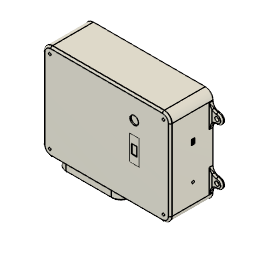
ROR Controller Housing v3 (Autodesk Fusion 360 design; units mm, degrees)
Autodesk Fusion 360 part; units mm, degrees
sketch "PCB Outline" plane through (0, 0, 0) normal (0, 0, 1) x (-1, 0, 0)
  line L0 (36.6395, 48.387) -> (-36.6395, 48.387) construction
  line L1 (-36.6395, 48.387) -> (-36.6395, -48.387) construction
  line L2 (-36.6395, -48.387) -> (36.6395, -48.387) construction
  line L3 (36.6395, -48.387) -> (36.6395, 48.387) construction
  line L4 (36.6395, 48.387) -> (-36.6395, -48.387) construction
  line L5 (-36.6395, 48.387) -> (36.6395, -48.387) construction
  line L6 (36.6395, 44.196) -> (-36.6395, 44.196) construction
  line L7 (33.5915, -48.387) -> (33.5915, 48.387) construction
  circle A0 centre (33.5915, 44.196) radius 1.5875 construction
  circle A1 centre (-32.9565, 44.196) radius 1.5875 construction
  circle A2 centre (33.5915, -44.196) radius 1.5875 construction
  circle A3 centre (-32.9565, -44.196) radius 1.5875 construction
  line L8 (-79.451, -48.75) -> (-59.451, -48.75) construction
  line L9 (-59.451, -48.75) -> (-59.451, 31.25) construction
  line L10 (-59.451, 31.25) -> (-79.451, 31.25) construction
  line L11 (-79.451, 31.25) -> (-79.451, -48.75) construction
  line L12 (-79.451, -48.75) -> (-59.451, 31.25) construction
  line L13 (-59.451, -48.75) -> (-79.451, 31.25) construction
  line L14 (-77.301, -46.625) -> (-61.601, -46.625) construction
  line L15 (-61.601, -46.625) -> (-61.601, 29.125) construction
  line L16 (-61.601, 29.125) -> (-77.301, 29.125) construction
  line L17 (-77.301, 29.125) -> (-77.301, -46.625) construction
  line L18 (-77.301, -46.625) -> (-61.601, 29.125) construction
  line L19 (-61.601, -46.625) -> (-77.301, 29.125) construction
  circle A4 centre (-77.301, -46.625) radius 1 construction
  circle A5 centre (-61.601, -46.625) radius 1 construction
  circle A6 centre (-77.301, 29.125) radius 1 construction
  circle A7 centre (-61.601, 29.125) radius 1 construction
  point P0 (-69.451, -8.75)
  point P1 (-69.451, -8.75)
  dimension "d1" = 73.279
  dimension "d2" = 96.774
  dimension "d3" = -4.191
  dimension "d4" = -3.048
  dimension "d5" = 3.175
  dimension "d8" = -66.548
  dimension "d9" = -88.392
  dimension "d11" = 70
  dimension "d12" = 20
  dimension "d13" = 80
  dimension "d14" = 15.7
  dimension "d15" = 75.75
  dimension "d16" = 2
  constraint horizontal L0
  constraint perpendicular L0 L1
  constraint parallel L0 L2
  constraint parallel L1 L3
  constraint coincident L4 origin
  constraint coincident L5 origin
  constraint coincident L7 A0.centre
  constraint coincident L6 A0.centre
  constraint horizontal L8
  constraint perpendicular L8 L9
  constraint parallel L8 L10
  constraint parallel L9 L11
  constraint coincident L12 P1
  constraint coincident L13 P1
  constraint horizontal L14
  constraint perpendicular L14 L15
  constraint parallel L14 L16
  constraint parallel L15 L17
  constraint coincident L18 P1
  constraint coincident L19 P1
  constraint coincident P1 P0
  constraint coincident L14.start L17.end
  constraint coincident L14.end L15.start
  constraint coincident L16.end L17.start
  constraint coincident L15.end L16.start
  constraint equal A4 A6
  constraint equal A4 A7
  constraint equal A4 A5
  measures "d1" distance of L1.end L2.end
  measures "d2" distance of L0.end L1.end
  measures "d5" diameter of A0
  measures "d11" distance of origin P1
  measures "d12" distance of L9.end L10.end
  measures "d13" distance of L8.end L9.end
  measures "d14" distance of L15.end L16.end
  measures "d15" distance of L14.end L15.end
  measures "d16" diameter of A4
other "Base Mesh Feature2"
other "MeshRepair2"
other "Modify2"
other "Modify3"
sketch "Base" plane through (0, 0, 0) normal (0, 0, 1) x (1, 0, 0)
  line L0 (-55, 57.5) -> (-55, -57.5)
  line L1 (-47.5, -65) -> (112.5, -65)
  line L2 (120, -57.5) -> (120, 57.5)
  line L3 (112.5, 65) -> (-47.5, 65)
  circle A0 centre (-33.5915, 44.196) radius 3.75
  circle A1 centre (32.9565, 44.196) radius 3.75
  circle A2 centre (32.9565, -44.196) radius 3.75
  circle A3 centre (-33.5915, -44.196) radius 3.75
  circle A4 centre (61.601, 46.625) radius 3.75
  circle A5 centre (77.301, 46.625) radius 3.75
  circle A6 centre (77.301, -29.125) radius 3.75
  circle A7 centre (61.601, -29.125) radius 3.75
  arc A8 (-47.5, 65) -> (-55, 57.5) centre (-47.5, 57.5) ccw
  arc A9 (120, 57.5) -> (112.5, 65) centre (112.5, 57.5) ccw
  arc A10 (112.5, -65) -> (120, -57.5) centre (112.5, -57.5) ccw
  arc A11 (-55, -57.5) -> (-47.5, -65) centre (-47.5, -57.5) ccw
  line L4 (-47.5, -68.5) -> (112.5, -68.5)
  arc A12 (112.5, -68.5) -> (123.5, -57.5) centre (112.5, -57.5) ccw
  line L5 (123.5, -57.5) -> (123.5, 57.5)
  arc A13 (123.5, 57.5) -> (112.5, 68.5) centre (112.5, 57.5) ccw
  line L6 (112.5, 68.5) -> (-47.5, 68.5)
  arc A14 (-47.5, 68.5) -> (-58.5, 57.5) centre (-47.5, 57.5) ccw
  line L7 (-58.5, 57.5) -> (-58.5, -57.5)
  arc A15 (-58.5, -57.5) -> (-47.5, -68.5) centre (-47.5, -57.5) ccw
  line L8 (-58.5, 0) -> (123.5, 0) construction
  line L9 (123.5, 0) -> (132.5, 0) construction
  line L10 (-58.5, 0) -> (-67.5, 0) construction
  line L11 (132.5, 0) -> (132.5, 40) construction
  line L12 (132.5, 0) -> (132.5, -40) construction
  line L13 (-67.5, 0) -> (-67.5, 40) construction
  line L14 (-67.5, 0) -> (-67.5, -40) construction
  circle A16 centre (-67.5, 40) radius 7.5
  circle A17 centre (-67.5, -40) radius 7.5
  circle A18 centre (132.5, -40) radius 7.5
  circle A19 centre (132.5, 40) radius 7.5
  line L15 (132.5, 32.5) -> (123.5, 32.5)
  line L16 (132.5, 47.5) -> (123.5, 47.5)
  line L17 (132.5, -32.5) -> (123.5, -32.5)
  line L18 (132.5, -47.5) -> (123.5, -47.5)
  line L19 (-67.5, -32.5) -> (-58.5, -32.5)
  line L20 (-67.5, -47.5) -> (-58.5, -47.5)
  line L21 (-67.5, 32.5) -> (-58.5, 32.5)
  line L22 (-67.5, 47.5) -> (-58.5, 47.5)
  point P0 (-33.5915, 44.196)
  point P1 (32.9565, 44.196)
  point P2 (32.9565, -44.196)
  point P3 (-33.5915, -44.196)
  point P4 (61.601, 46.625)
  point P5 (77.301, 46.625)
  point P6 (77.301, -29.125)
  point P7 (61.601, -29.125)
  dimension "d10" = 7.5
  dimension "d17" = 7.5
  dimension "d18" = 7.5
  dimension "d19" = 3.5
  dimension "d116" = 9
  dimension "d118" = 40
  dimension "d119" = 15
  constraint perpendicular L0 L1
  constraint parallel L0 L2
  constraint parallel L1 L3
  constraint vertical L0
  constraint coincident P0 A0.centre
  constraint coincident P1 A1.centre
  constraint coincident P2 A2.centre
  constraint coincident P3 A3.centre
  constraint equal A0 A1
  constraint equal A0 A3
  constraint equal A0 A2
  constraint coincident P4 A4.centre
  constraint coincident P5 A5.centre
  constraint coincident P6 A6.centre
  constraint coincident P7 A7.centre
  constraint equal A4 A5
  constraint equal A4 A6
  constraint equal A4 A7
  constraint tangent L0 A8
  constraint tangent L3 A8
  constraint tangent L3 A9
  constraint tangent L2 A9
  constraint equal A8 A9
  constraint tangent L2 A10
  constraint tangent L1 A10
  constraint equal A8 A10
  constraint tangent L1 A11
  constraint tangent L0 A11
  constraint equal A8 A11
  constraint midpoint L7 L8.start
  constraint midpoint L5 L8.end
  constraint perpendicular L5 L9
  constraint perpendicular L7 L10
  constraint perpendicular L9 L11
  constraint perpendicular L9 L12
  constraint perpendicular L10 L13
  constraint perpendicular L10 L14
  constraint equal L11 L12
  constraint equal L13 L14
  constraint equal L9 L10
  constraint coincident L13.end A16.centre
  constraint coincident L14.end A17.centre
  constraint coincident L12.end A18.centre
  constraint coincident L11.end A19.centre
  constraint equal A16 A19
  constraint equal A16 A18
  constraint equal A16 A17
  constraint coincident A19 L15.start
  constraint coincident L11 L15.start
  constraint coincident L5 L15.end
  constraint tangent A19 L15
  constraint coincident A19 L16.start
  constraint coincident L5 L16.end
  constraint tangent A19 L16
  constraint perpendicular L5 L16
  constraint coincident L12 L17.start
  constraint coincident A18 L17.start
  constraint coincident L5 L17.end
  constraint tangent A18 L17
  constraint coincident A18 L18.start
  constraint coincident L5 L18.end
  constraint tangent A18 L18
  constraint perpendicular L5 L18
  constraint coincident A17 L19.start
  constraint coincident L14 L19.start
  constraint coincident L7 L19.end
  constraint tangent A17 L19
  constraint coincident A17 L20.start
  constraint coincident L7 L20.end
  constraint tangent A17 L20
  constraint perpendicular L7 L20
  constraint coincident A16 L21.start
  constraint coincident L13 L21.start
  constraint coincident L7 L21.end
  constraint tangent A16 L21
  constraint coincident A16 L22.start
  constraint coincident L7 L22.end
  constraint tangent A16 L22
  constraint perpendicular L7 L22
  measures "d10" diameter of A0
  measures "d17" diameter of A4
  measures "d18" radius of A8
  measures "d116" distance of L8.end L9.end
  measures "d118" distance of L9.end L11.end
  measures "d119" diameter of A16
extrude "Extrude1" add sketch "Base" against normal blind 3.5 contours L0 L1 L2 L3 A8 A9 A10 A11 | A0 | A1 | A2 | A3 | A4 | A5 | A6 | A7 | L4 A12 L5 A13 L6 A14 L7 A15 makes body 1
extrude "Extrude2" add sketch "Base" along normal blind 10 contours A0 | A1 | A2 | A3 | A4 | A5 | A6 | A7 bodies 1
sketch "Board Mounting Holes" plane through (0, 0, 10) normal (0, 0, 1) x (1, 0, 0)
  circle A0 centre (-33.5915, 44.196) radius 3.75
  point P0 (-33.5915, 44.196)
  point P1 (32.9565, 44.196)
  point P2 (32.9565, -44.196)
  point P3 (-33.5915, -44.196)
  point P4 (61.601, -29.125)
  point P5 (77.301, -29.125)
  point P6 (61.601, 46.625)
  point P7 (77.301, 46.625)
hole "Hole1" at (61.601, 46.625, 10) at (77.301, 46.625, 10) at (61.601, -29.125, 10) at (77.301, -29.125, 10) direction (0, 0, -1) diameter 3.8 depth 5 tip angle 180 bodies 1
hole "Hole2" at (-33.5915, 44.196, 10) at (-33.5915, -44.196, 10) at (32.9565, -44.196, 10) at (32.9565, 44.196, 10) direction (0, 0, -1) diameter 3.5 depth 5 tip angle 180 bodies 1
extrude "Extrude3" add sketch "Base" along normal blind 55 contours L4 A12 L5 A13 L6 A14 L7 A15 bodies 1
ref_plane "WorkPlane1" through (32.5, 0, 53) normal (0, 0, 1) x (1, 0, 0)
sketch "Lid Supports" plane through (0, 0, 53) normal (0, 0, 1) x (1, 0, 0)
  line L0 (-55, 57.5) -> (-55, -57.5)
  arc A0 (-55, -57.5) -> (-47.5, -65) centre (-47.5, -57.5) ccw
  line L1 (-47.5, -65) -> (112.5, -65)
  arc A1 (112.5, -65) -> (120, -57.5) centre (112.5, -57.5) ccw
  arc A2 (120, 57.5) -> (112.5, 65) centre (112.5, 57.5) ccw
  arc A3 (-47.5, 65) -> (-55, 57.5) centre (-47.5, 57.5) ccw
  line L2 (112.5, 65) -> (-47.5, 65)
  line L3 (120, -57.5) -> (120, 57.5)
  line L4 (-20, 65) -> (85, 65)
  line L5 (120, 30) -> (120, -30)
  line L6 (85, -65) -> (-20, -65)
  line L7 (-55, -30) -> (-55, 30)
  arc A4 (-20, 65) -> (-55, 30) centre (-20, 30) ccw
  arc A5 (120, 30) -> (85, 65) centre (85, 30) ccw
  arc A6 (85, -65) -> (120, -30) centre (85, -30) ccw
  arc A7 (-55, -30) -> (-20, -65) centre (-20, -30) ccw
  line L8 (-52.8033, 62.8033) -> (-44.7487, 54.7487) construction
  line L9 (-52.8033, -62.8033) -> (-44.7487, -54.7487) construction
  line L10 (117.8033, 62.8033) -> (109.7487, 54.7487) construction
  line L11 (117.8033, -62.8033) -> (109.7487, -54.7487) construction
  point P0 (-48.776, 58.776)
  point P1 (-48.776, -58.776)
  point P2 (113.776, -58.776)
  point P3 (113.776, 58.776)
  dimension "d33" = 35
  constraint horizontal L4
  constraint vertical L5
  constraint horizontal L6
  constraint vertical L7
  constraint tangent L4 A4
  constraint tangent L7 A4
  constraint tangent L4 A5
  constraint tangent L5 A5
  constraint equal A4 A5
  constraint tangent L5 A6
  constraint tangent L6 A6
  constraint equal A4 A6
  constraint tangent L6 A7
  constraint tangent L7 A7
  constraint equal A4 A7
  constraint midpoint A3 L8.start
  constraint midpoint A4 L8.end
  constraint midpoint L8 P0
  constraint midpoint A0 L9.start
  constraint midpoint A7 L9.end
  constraint midpoint A2 L10.start
  constraint midpoint A5 L10.end
  constraint midpoint A1 L11.start
  constraint midpoint A6 L11.end
  constraint midpoint L9 P1
  constraint midpoint L11 P2
  constraint midpoint L10 P3
  measures "d33" radius of A4
extrude "Extrude4" add sketch "Lid Supports" against normal blind 10 contours L0 A3 L2 A4 | L0 A0 L1 A7 | A2 L2 L3 A5 | L1 A1 L3 A6 bodies 1
hole "Hole3" at (-48.776, 58.776, 53) at (-48.776, -58.776, 53) at (113.776, -58.776, 53) at (113.776, 58.776, 53) direction (0, 0, -1) diameter 3.5 depth 10 tip angle 180 counterbore diameter 4.9 counterbore depth 4 bodies 1
sketch "Bottom Protrusion" plane through (0, -68.5, 0) normal (0, -1, 0) x (1, 0, 0)
  line L0 (-47.5, 55) -> (-47.5, -3.5)
  line L1 (-47.5, -3.5) -> (112.5, -3.5)
  line L2 (112.5, -3.5) -> (112.5, 55)
  line L3 (112.5, 55) -> (-47.5, 55)
  line L4 (32.5, 47.5) -> (-32.5, 47.5)
  line L5 (-42.5, 37.5) -> (-42.5, 12.5)
  line L6 (-32.5, 2.5) -> (32.5, 2.5)
  line L7 (42.5, 12.5) -> (42.5, 37.5)
  line L8 (42.5, 47.5) -> (-42.5, 2.5) construction
  line L9 (-42.5, 47.5) -> (42.5, 2.5) construction
  arc A0 (-32.5, 47.5) -> (-42.5, 37.5) centre (-32.5, 37.5) ccw
  arc A1 (42.5, 37.5) -> (32.5, 47.5) centre (32.5, 37.5) ccw
  arc A2 (32.5, 2.5) -> (42.5, 12.5) centre (32.5, 12.5) ccw
  arc A3 (-42.5, 12.5) -> (-32.5, 2.5) centre (-32.5, 12.5) ccw
  line L10 (-32.5, -1) -> (32.5, -1)
  arc A4 (32.5, -1) -> (46, 12.5) centre (32.5, 12.5) ccw
  line L11 (46, 12.5) -> (46, 37.5)
  arc A5 (46, 37.5) -> (32.5, 51) centre (32.5, 37.5) ccw
  line L12 (32.5, 51) -> (-32.5, 51)
  arc A6 (-32.5, 51) -> (-46, 37.5) centre (-32.5, 37.5) ccw
  line L13 (-46, 37.5) -> (-46, 12.5)
  arc A7 (-46, 12.5) -> (-32.5, -1) centre (-32.5, 12.5) ccw
  point P0 (0, 25)
  dimension "d39" = 85
  dimension "d40" = 45
  dimension "d41" = 10
  dimension "d42" = 3.5
  constraint horizontal L4
  constraint perpendicular L4 L5
  constraint parallel L4 L6
  constraint parallel L5 L7
  constraint coincident L8 P0
  constraint coincident L9 P0
  constraint coincident L9.start L4
  constraint coincident L9.start L5
  constraint tangent L4 A0
  constraint tangent L5 A0
  constraint coincident L8.start L4
  constraint coincident L8.start L7
  constraint tangent L4 A1
  constraint tangent L7 A1
  constraint equal A0 A1
  constraint coincident L9.end L7
  constraint coincident L9.end L6
  constraint tangent L7 A2
  constraint tangent L6 A2
  constraint equal A0 A2
  constraint coincident L8.end L6
  constraint coincident L8.end L5
  constraint tangent L6 A3
  constraint tangent L5 A3
  constraint equal A0 A3
  measures "d39" distance of L8.end L9.end
  measures "d40" distance of L9.start L8.end
  measures "d41" radius of A0
extrude "Extrude5" add sketch "Bottom Protrusion" along normal blind 15 contours L4 L5 L6 L7 A0 A1 A2 A3 | L10 A4 L11 A5 L12 A6 L13 A7 bodies 1
extrude "Extrude6" cut sketch "Bottom Protrusion" against normal blind 3.5 contours L4 L5 L6 L7 A0 A1 A2 A3 bodies 1
extrude "Extrude7" cut sketch "Bottom Protrusion" along normal blind 12.5 contours L4 L5 L6 L7 A0 A1 A2 A3 bodies 1
sketch "Cable Ports" plane through (0, -83.5, 0) normal (0, -1, 0) x (1, 0, 0)
  arc A0 (-46, 12.5) -> (-32.5, -1) centre (-32.5, 12.5) ccw
  line L0 (-32.5, -1) -> (32.5, -1)
  arc A1 (32.5, -1) -> (46, 12.5) centre (32.5, 12.5) ccw
  line L1 (46, 12.5) -> (46, 37.5)
  arc A2 (46, 37.5) -> (32.5, 51) centre (32.5, 37.5) ccw
  line L2 (32.5, 51) -> (-32.5, 51)
  arc A3 (-32.5, 51) -> (-46, 37.5) centre (-32.5, 37.5) ccw
  line L3 (-46, 37.5) -> (-46, 12.5)
  line L4 (-46, 25) -> (46, 25) construction
  line L5 (0, 51) -> (0, -1) construction
  line L6 (-17.5, 51) -> (-17.5, -1) construction
  line L7 (17.5, 51) -> (17.5, -1) construction
  point P0 (-17.5, 25)
  point P1 (17.5, 25)
  dimension "d49" = 17.5
  dimension "d50" = -17.5
  constraint midpoint L3 L4.start
  constraint midpoint L1 L4.end
  constraint midpoint L2 L5.start
  constraint midpoint L0 L5.end
  constraint midpoint L6 P0
  constraint midpoint L7 P1
hole "Hole4" at (17.5, -83.5, 25) at (-17.5, -83.5, 25) direction (0, 1, 0) diameter 22.5 depth 3.5 tip angle 180 bodies 1
fillet "Fillet1" radius 2 8 edges at (-46, -83.5, 25) (-42.0459, -83.5, 2.9541) (0, -83.5, -1) (42.0459, -83.5, 2.9541) (46, -83.5, 25) (42.0459, -83.5, 47.0459) (0, -83.5, 51) (-42.0459, -83.5, 47.0459) on bodies 1
fillet "Fillet2" radius 2 8 edges at (46, -68.5, 25) (42.0459, -68.5, 2.9541) (0, -68.5, -1) (-42.0459, -68.5, 2.9541) (-46, -68.5, 25) (-42.0459, -68.5, 47.0459) (0, -68.5, 51) (42.0459, -68.5, 47.0459) on bodies 1
sketch "Park Sensor Jacks" plane through (0, -65, 0) normal (0, -1, 0) x (1, 0, 0)
  arc A0 (-32.5, 53) -> (-47.5, 41.4051) centre (-32.5, 37.5) ccw
  line L0 (-32.5, 53) -> (32.5, 53)
  arc A1 (48, 37.5) -> (32.5, 53) centre (32.5, 37.5) ccw
  line L1 (48, 37.5) -> (48, 12.5)
  arc A2 (32.5, -3) -> (48, 12.5) centre (32.5, 12.5) ccw
  line L2 (32.5, -3) -> (-32.5, -3)
  arc A3 (-47.5, 8.5949) -> (-32.5, -3) centre (-32.5, 12.5) ccw
  line L3 (-47.5, 8.5949) -> (-47.5, -3.5)
  line L4 (-47.5, -3.5) -> (112.5, -3.5)
  line L5 (112.5, -3.5) -> (112.5, 55)
  line L6 (112.5, 55) -> (-47.5, 55)
  line L7 (-47.5, 55) -> (-47.5, 41.4051)
  line L8 (70, 0) -> (90, 0) construction
  line L9 (80, 0) -> (80, 15) construction
  line L10 (80, 15) -> (90, 15) construction
  line L11 (80, 15) -> (70, 15) construction
  line L12 (32.5, 47.5) -> (-20, 47.5)
  line L13 (-20, 47.5) -> (-20, 53)
  line L14 (-20, 53) -> (-47.5, 53)
  line L15 (-47.5, 53) -> (-47.5, 55)
  line L16 (-47.5, 55) -> (112.5, 55)
  line L17 (112.5, 55) -> (112.5, 53)
  line L18 (112.5, 53) -> (85, 53)
  line L19 (85, 53) -> (85, 43)
  line L20 (85, 43) -> (112.5, 43)
  line L21 (112.5, 43) -> (112.5, 0)
  line L22 (112.5, 0) -> (-47.5, 0)
  line L23 (-47.5, 0) -> (-47.5, 43)
  line L24 (-47.5, 43) -> (-40.8516, 43)
  arc A4 (-40.8516, 43) -> (-42.5, 37.5) centre (-32.5, 37.5) ccw
  line L25 (-42.5, 37.5) -> (-42.5, 12.5)
  arc A5 (-42.5, 12.5) -> (-32.5, 2.5) centre (-32.5, 12.5) ccw
  line L26 (-32.5, 2.5) -> (32.5, 2.5)
  arc A6 (32.5, 2.5) -> (42.5, 12.5) centre (32.5, 12.5) ccw
  line L27 (42.5, 12.5) -> (42.5, 37.5)
  arc A7 (42.5, 37.5) -> (32.5, 47.5) centre (32.5, 37.5) ccw
  line L28 (80, 0) -> (80, 30)
  line L29 (87.2, 35.65) -> (72.8, 35.65)
  line L30 (72.8, 35.65) -> (72.8, 24.35)
  line L31 (72.8, 24.35) -> (87.2, 24.35)
  line L32 (87.2, 24.35) -> (87.2, 35.65)
  line L33 (87.2, 35.65) -> (72.8, 24.35) construction
  line L34 (72.8, 35.65) -> (87.2, 24.35) construction
  circle A8 centre (70, 15) radius 4.15
  circle A9 centre (90, 15) radius 4.15
  point P0 (80, 0)
  point P1 (80, 30)
  dimension "d58" = 15
  dimension "d59" = 10
  dimension "d65" = 30
  dimension "d69" = 14.4
  dimension "d70" = 11.3
  dimension "d71" = 8.3
  constraint coincident P0 L9.start
  constraint perpendicular L8 L9
  constraint perpendicular L9 L10
  constraint perpendicular L9 L11
  constraint equal L10 L11
  constraint perpendicular L8 L28
  constraint horizontal L29
  constraint perpendicular L29 L30
  constraint parallel L29 L31
  constraint parallel L30 L32
  constraint coincident L33 P1
  constraint coincident L34 P1
  constraint coincident P1 L28.end
  constraint coincident L11.end A8.centre
  constraint coincident L10.end A9.centre
  constraint equal A8 A9
  measures "d58" distance of P0 L9.end
  measures "d59" distance of L9.end L10.end
  measures "d65" distance of P0 P1
  measures "d69" distance of L30.end L31.end
  measures "d70" distance of L29.end L30.end
  measures "d71" diameter of A8
hole "Hole5" at (70, -65, 15) at (90, -65, 15) direction (0, -1, 0) diameter 6 depth 3.5 tip angle 180 counterbore diameter 12 counterbore depth 1.5 bodies 1
hole "Hole6" at (80, -65, 30) direction (0, -1, 0) diameter 10 depth 3.5 tip angle 180 bodies 1
extrude "Extrude8" add sketch "Park Sensor Jacks" against normal blind 27 separate body contours L29 L30 L31 L32 makes body 2
extrude "Extrude9" add sketch "Park Sensor Jacks" against normal blind 20 separate body contours A8 | A9 makes body 3 at (74.1448, -51.6667, 14.7931) makes body 4 at (94.1448, -51.6667, 14.7931)
sketch "Bypass Switch and Power LED" plane through (120, 0, 0) normal (-1, 0, 0) x (0, 0, 1)
  line L0 (43, 30) -> (43, 57.5)
  line L1 (43, 57.5) -> (0, 57.5)
  line L2 (0, 57.5) -> (0, -57.5)
  line L3 (0, -57.5) -> (43, -57.5)
  line L4 (43, -57.5) -> (43, -30)
  line L5 (43, -30) -> (53, -30)
  line L6 (53, -30) -> (53, -57.5)
  line L7 (53, -57.5) -> (55, -57.5)
  line L8 (55, -57.5) -> (55, 57.5)
  line L9 (55, 57.5) -> (53, 57.5)
  line L10 (53, 57.5) -> (53, 30)
  line L11 (53, 30) -> (43, 30)
  line L12 (0, 20) -> (25, 20) construction
  line L13 (28.25, 29.75) -> (21.75, 29.75)
  line L14 (21.75, 29.75) -> (21.75, 10.25)
  line L15 (21.75, 10.25) -> (28.25, 10.25)
  line L16 (28.25, 10.25) -> (28.25, 29.75)
  line L17 (28.25, 29.75) -> (21.75, 10.25) construction
  line L18 (21.75, 29.75) -> (28.25, 10.25) construction
  line L19 (27.25, 23.75) -> (22.75, 23.75)
  line L20 (22.75, 23.75) -> (22.75, 16.25)
  line L21 (22.75, 16.25) -> (27.25, 16.25)
  line L22 (27.25, 16.25) -> (27.25, 23.75)
  line L23 (27.25, 23.75) -> (22.75, 16.25) construction
  line L24 (22.75, 23.75) -> (27.25, 16.25) construction
  line L25 (25, 20) -> (25, -30) construction
  point P0 (25, 20)
  point P1 (25, 20)
  dimension "d76" = 25
  dimension "d77" = 6.5
  dimension "d78" = 19.5
  dimension "d79" = 4.5
  dimension "d80" = 7.5
  constraint coincident L2 L12.start
  constraint perpendicular L8 L12
  constraint horizontal L13
  constraint perpendicular L13 L14
  constraint parallel L13 L15
  constraint parallel L14 L16
  constraint coincident L17 P1
  constraint coincident L18 P1
  constraint coincident P1 P0
  constraint horizontal L19
  constraint perpendicular L19 L20
  constraint parallel L19 L21
  constraint parallel L20 L22
  constraint coincident L23 P1
  constraint coincident L24 P1
  constraint parallel L8 L25
  measures "d76" distance of L12.start P1
  measures "d77" distance of L14.end L15.end
  measures "d78" distance of L13.end L14.end
  measures "d79" distance of L20.end L21.end
  measures "d80" distance of L19.end L20.end
extrude "Extrude10" cut sketch "Bypass Switch and Power LED" against normal blind 3.5 contours L19 L20 L21 L22 bodies 1
extrude "Extrude11" cut sketch "Bypass Switch and Power LED" against normal blind 2 contours L13 L14 L15 L16 bodies 1
ref_plane "WorkPlane2" through (32.5, 0, 55) normal (0, 0, 1) x (1, 0, 0)
sketch "Lid" plane through (0, 0, 55) normal (0, 0, 1) x (1, 0, 0)
  arc A0 (-55, -57.5) -> (-47.5, -65) centre (-47.5, -57.5) ccw
  line L0 (-55, -57.5) -> (-55, 57.5)
  arc A1 (-47.5, 65) -> (-55, 57.5) centre (-47.5, 57.5) ccw
  line L1 (-47.5, 65) -> (112.5, 65)
  arc A2 (120, 57.5) -> (112.5, 65) centre (112.5, 57.5) ccw
  line L2 (120, 57.5) -> (120, -57.5)
  arc A3 (112.5, -65) -> (120, -57.5) centre (112.5, -57.5) ccw
  line L3 (112.5, -65) -> (-47.5, -65)
  arc A4 (-58.5, -57.5) -> (-47.5, -68.5) centre (-47.5, -57.5) ccw
  line L4 (-47.5, -68.5) -> (112.5, -68.5)
  arc A5 (112.5, -68.5) -> (123.5, -57.5) centre (112.5, -57.5) ccw
  line L5 (123.5, -57.5) -> (123.5, 57.5)
  arc A6 (123.5, 57.5) -> (112.5, 68.5) centre (112.5, 57.5) ccw
  line L6 (112.5, 68.5) -> (-47.5, 68.5)
  arc A7 (-47.5, 68.5) -> (-58.5, 57.5) centre (-47.5, 57.5) ccw
  line L7 (-58.5, 57.5) -> (-58.5, -57.5)
  arc A8 (-55, -57.5) -> (-47.5, -65) centre (-47.5, -57.5) ccw construction
  line L8 (-47.5, -65) -> (-20, -65) construction
  arc A9 (-55, -30) -> (-20, -65) centre (-20, -30) ccw construction
  line L9 (-55, -30) -> (-55, -57.5) construction
  arc A10 (-47.5, 65) -> (-55, 57.5) centre (-47.5, 57.5) ccw construction
  line L10 (-55, 57.5) -> (-55, 30) construction
  arc A11 (-20, 65) -> (-55, 30) centre (-20, 30) ccw construction
  line L11 (-20, 65) -> (-47.5, 65) construction
  arc A12 (112.5, -65) -> (120, -57.5) centre (112.5, -57.5) ccw construction
  line L12 (120, -57.5) -> (120, -30) construction
  arc A13 (85, -65) -> (120, -30) centre (85, -30) ccw construction
  line L13 (85, -65) -> (112.5, -65) construction
  arc A14 (120, 57.5) -> (112.5, 65) centre (112.5, 57.5) ccw construction
  line L14 (112.5, 65) -> (85, 65) construction
  arc A15 (120, 30) -> (85, 65) centre (85, 30) ccw construction
  line L15 (120, 30) -> (120, 57.5) construction
  circle A16 centre (-48.776, -58.776) radius 2.45
  circle A17 centre (-48.776, 58.776) radius 2.45
  circle A18 centre (113.776, -58.776) radius 2.45
  circle A19 centre (113.776, 58.776) radius 2.45
  point P0 (-48.776, 58.776)
  point P1 (-48.776, -58.776)
  point P2 (113.776, -58.776)
  point P3 (113.776, 58.776)
extrude "Extrude12" add sketch "Lid" along normal blind 2.75 separate body contours A0 L0 A1 L1 A2 L2 A3 L3 | A4 L4 A5 L5 A6 L6 A7 L7 | A16 | A17 | A18 | A19 makes body 5
fillet "Fillet3" radius 2.5 8 edges at (32.5, -68.5, 57.75) (120.2782, -65.2782, 57.75) (123.5, 0, 57.75) (120.2782, 65.2782, 57.75) (32.5, 68.5, 57.75) (-55.2782, 65.2782, 57.75) (-58.5, 0, 57.75) (-55.2782, -65.2782, 57.75) on bodies 5
extrude "Extrude13" add sketch "Lid" against normal blind 1.75 thin wall 3 inside contours A0 L0 A1 L1 A2 L2 A3 L3 | A16 | A17 | A18 | A19 bodies 5
move_face "OffsetFaces1" offset -0.25 8 faces at (117.1362, 63.3954, 53.8333) (5.8333, 65, 54.4167) (120, 19.1667, 54.4167) (116.25, -63.9952, 53.8333) (59.1667, -65, 54.4167) (-55, -19.1667, 54.4167) (-54.4628, -60.2875, 53.8333) (-50.2875, 64.4628, 53.8333) on bodies 5
sketch "Lid Screw Holes" plane through (0, 0, 57.75) normal (0, 0, 1) x (1, 0, 0)
  line L0 (-47.5, -66) -> (112.5, -66)
  arc A0 (112.5, -66) -> (121, -57.5) centre (112.5, -57.5) ccw
  line L1 (121, -57.5) -> (121, 57.5)
  arc A1 (121, 57.5) -> (112.5, 66) centre (112.5, 57.5) ccw
  line L2 (112.5, 66) -> (-47.5, 66)
  arc A2 (-47.5, 66) -> (-56, 57.5) centre (-47.5, 57.5) ccw
  line L3 (-56, 57.5) -> (-56, -57.5)
  arc A3 (-56, -57.5) -> (-47.5, -66) centre (-47.5, -57.5) ccw
  circle A4 centre (113.776, 58.776) radius 2.45
  arc A5 (120, 57.5) -> (112.5, 65) centre (112.5, 57.5) ccw
  line L4 (112.5, 65) -> (85, 65)
  arc A6 (120, 30) -> (85, 65) centre (85, 30) ccw
  line L5 (120, 30) -> (120, 57.5)
  circle A7 centre (113.776, -58.776) radius 2.45
  arc A8 (112.5, -65) -> (120, -57.5) centre (112.5, -57.5) ccw
  line L6 (120, -57.5) -> (120, -30)
  arc A9 (85, -65) -> (120, -30) centre (85, -30) ccw
  line L7 (85, -65) -> (112.5, -65)
  circle A10 centre (-48.776, -58.776) radius 2.45
  arc A11 (-55, -57.5) -> (-47.5, -65) centre (-47.5, -57.5) ccw
  line L8 (-47.5, -65) -> (-20, -65)
  arc A12 (-55, -30) -> (-20, -65) centre (-20, -30) ccw
  line L9 (-55, -30) -> (-55, -57.5)
  circle A13 centre (-48.776, 58.776) radius 2.45
  arc A14 (-47.5, 65) -> (-55, 57.5) centre (-47.5, 57.5) ccw
  line L10 (-55, 57.5) -> (-55, 30)
  arc A15 (-20, 65) -> (-55, 30) centre (-20, 30) ccw
  line L11 (-20, 65) -> (-47.5, 65)
hole "Hole7" at (-48.776, -58.776, 57.75) at (-48.776, 58.776, 57.75) at (113.776, 58.776, 57.75) at (113.776, -58.776, 57.75) direction (0, 0, -1) diameter 3.5 depth 3.5 tip angle 180 bodies 5
sketch "Power Switch and Push Button" plane through (0, 0, 55) normal (0, 0, -1) x (-1, 0, 0)
  line L0 (47.5, 62) -> (-112.5, 62)
  arc A0 (-112.5, 62) -> (-117, 57.5) centre (-112.5, 57.5) ccw
  line L1 (-117, 57.5) -> (-117, -57.5)
  arc A1 (-117, -57.5) -> (-112.5, -62) centre (-112.5, -57.5) ccw
  line L2 (-112.5, -62) -> (47.5, -62)
  arc A2 (47.5, -62) -> (52, -57.5) centre (47.5, -57.5) ccw
  line L3 (52, -57.5) -> (52, 57.5)
  arc A3 (52, 57.5) -> (47.5, 62) centre (47.5, 57.5) ccw
  line L4 (47.5, 37) -> (-112.5, 37) construction
  line L5 (47.5, 0) -> (-112.5, 0) construction
  line L6 (-72, 57.5) -> (-72, -57.5) construction
  line L7 (-65.25, -17.75) -> (-78.75, -17.75)
  line L8 (-78.75, -17.75) -> (-78.75, 17.75)
  line L9 (-78.75, 17.75) -> (-65.25, 17.75)
  line L10 (-65.25, 17.75) -> (-65.25, -17.75)
  line L11 (-65.25, -17.75) -> (-78.75, 17.75) construction
  line L12 (-78.75, -17.75) -> (-65.25, 17.75) construction
  line L13 (-68.25, -6.5) -> (-75.75, -6.5)
  line L14 (-75.75, -6.5) -> (-75.75, 6.5)
  line L15 (-75.75, 6.5) -> (-68.25, 6.5)
  line L16 (-68.25, 6.5) -> (-68.25, -6.5)
  line L17 (-68.25, -6.5) -> (-75.75, 6.5) construction
  line L18 (-75.75, -6.5) -> (-68.25, 6.5) construction
  circle A4 centre (-72, 37) radius 6.125 construction
  circle A5 centre (-113.776, 58.776) radius 1.75
  circle A6 centre (48.776, -58.776) radius 1.75
  circle A7 centre (48.776, 58.776) radius 1.75
  circle A8 centre (-113.776, -58.776) radius 1.75
  arc A9 (20, -65) -> (55, -30) centre (20, -30) ccw
  arc A10 (55, 30) -> (20, 65) centre (20, 30) ccw
  arc A11 (-120, -30) -> (-85, -65) centre (-85, -30) ccw
  arc A12 (-85, 65) -> (-120, 30) centre (-85, 30) ccw
  point P0 (-72, 37)
  point P1 (-72, 0)
  point P2 (-72, 0)
  point P3 (-72, 0)
  dimension "d99" = -25
  dimension "d100" = -62
  dimension "d101" = -45
  dimension "d102" = 13.5
  dimension "d103" = 35.5
  dimension "d104" = 7.5
  dimension "d105" = 13
  dimension "d106" = 12.25
  constraint coincident L4 P0
  constraint coincident L6 P0
  constraint coincident L5 P3
  constraint coincident L6 P3
  constraint horizontal L7
  constraint perpendicular L7 L8
  constraint parallel L7 L9
  constraint parallel L8 L10
  constraint coincident L11 P3
  constraint coincident L12 P3
  constraint coincident P3 P2
  constraint horizontal L13
  constraint perpendicular L13 L14
  constraint parallel L13 L15
  constraint parallel L14 L16
  constraint coincident L17 P3
  constraint coincident L18 P3
  constraint coincident P0 A4.centre
  measures "d102" distance of L8.end L9.end
  measures "d103" distance of L7.end L8.end
  measures "d104" distance of L14.end L15.end
  measures "d105" distance of L13.end L14.end
  measures "d106" diameter of A4
extrude "Extrude14" cut sketch "Power Switch and Push Button" against normal blind 3.5 contours L13 L14 L15 L16 bodies 5
extrude "Extrude15" cut sketch "Power Switch and Push Button" against normal blind 2 contours L7 L8 L9 L10 bodies 5
hole "Hole8" at (72, 37, 55) direction (0, 0, 1) diameter 12.25 depth 3.5 tip angle 180 counterbore diameter 27.5 counterbore depth 1 bodies 5
extrude "Extrude16" add sketch "Base" against normal blind 3.5 contours L7 A17 L19 L20 | L5 A18 L17 L18 | A17 | A18 | L7 A16 L21 L22 | L5 A19 L15 L16 | A16 | A19 bodies 1
fillet "Fillet4" radius 9 8 edges at (-58.5, -47.5, -1.75) (-58.5, 32.5, -1.75) (-58.5, -32.5, -1.75) (-58.5, 47.5, -1.75) (123.5, 47.5, -1.75) (123.5, -32.5, -1.75) (123.5, -47.5, -1.75) (123.5, 32.5, -1.75) on bodies 1
fillet "Fillet5" radius 2 4 edges at (123.5, -40, 0) (123.5, 40, 0) (-58.5, -40, 0) (-58.5, 40, 0) on bodies 1
hole "Hole9" at (-67.5, -40, 0) at (132.5, -40, 0) at (132.5, 40, 0) at (-67.5, 40, 0) direction (0, 0, -1) diameter 6 depth 3.5 tip angle 180 bodies 1
fillet "Fillet6" radius 2 20 edges at (-58.9936, -26.4397, 0.6844) (-63.6213, -31.6213, 0) (-75, -40, 0) (-63.6213, -48.3787, 0) (-58.9936, -53.5603, 0.6844) (-58.9936, 53.5603, 0.6844) (-63.6213, 48.3787, 0) (-75, 40, 0) (-63.6213, 31.6213, 0) (-58.9936, 26.4397, 0.6844) (123.9936, -53.5603, 0.6844) (128.6213, -48.3787, 0) (140, -40, 0) (128.6213, -31.6213, 0) (123.9936, -26.4397, 0.6844) (123.9936, 26.4397, 0.6844) (128.6213, 31.6213, 0) (140, 40, 0) (128.6213, 48.3787, 0) (123.9936, 53.5603, 0.6844) on bodies 1
hole "Hole10" at (120, -30, 25) direction (1, 0, 0) diameter 3.65 depth 4.5 tip angle 180 counterbore diameter 5.2 counterbore depth 1 bodies 1
extrude "Extrude17" add sketch "Power Switch and Push Button" along normal blind 1.75 contours L0 L3 A3 A10 | L0 A0 L1 A12 | L2 A2 L3 A9 | L1 A1 L2 A11 bodies 5
equation "d47 = 15 mm - 2.5 mm"
equation "d49 = ( 35 / 2 ) * 1 mm"
named bodies: "Housing Body", "Power Plug", "Park Jack 1", "Park Jack 2", "Lid"
